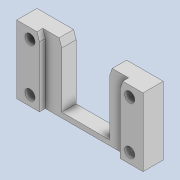
# Autodesk Inventor part: 0008-10-003
Saved by Autodesk Inventor 2020 (Build 240168000, 168)
## iProperties
Created: 2021-02-20
Part Number: 0008-10-003
Material: Generic
Document SubType Name: Modeling
Designer: Iulian Bors
Density: 1 g/cm^3
Appearance: Default
Mass: 4.90136 g
Surface Area: 35.6729 cm^2
Volume: 4.90136 cm^3
Description: Fixare Cap seringa
Author: Iulian Bors
Subject: 003
Autodesk Inventor part; units mm, degrees
ref_plane "YZ Plane" through (0, 0, 0) normal (1, 0, 0) x (0, 1, 0)
ref_plane "XZ Plane" through (0, 0, 0) normal (0, 1, 0) x (-1, 0, 0)
ref_plane "XY Plane" through (0, 0, 0) normal (0, 0, 1) x (1, 0, 0)
sketch "Sketch1" plane through (0, 0, 0) normal (0, 0, 1) x (1, 0, 0)
  line L0 (-25, 13.5) -> (25, 13.5)
  line L1 (25, 13.5) -> (25, -13.5)
  line L2 (25, -13.5) -> (-25, -13.5)
  line L3 (-25, -13.5) -> (-25, 13.5)
  point P0 (0, 0)
  point P1 (0, 13.5)
  point P2 (-25, 0)
  dimension "d0" = 27
  dimension "d1" = 50
  constraints: 8 end point, 2 midpoint, 2 parallel, 1 horizontal, 1 horizontal alignment, 1 perpendicular, 1 vertical alignment
  measures "d0" distance of L2.end L0.start
  measures "d1" distance of L0.start L0.end
extrude "Extrusion1" add sketch "Sketch1" along normal blind 8
sketch "Sketch2" plane through (0, 0, 8) normal (0, 0, 1) x (1, 0, 0)
  arc A0 (-10.3042, 3.1624) -> (-9.6648, 2.3936) centre (-9.9845, 2.778) ccw
  line L0 (-1.0786, 10.8363) -> (-10.3042, 3.1624)
  arc A1 (-0.4391, 10.0675) -> (-1.0786, 10.8363) centre (-0.7589, 10.4519) ccw
  line L1 (-9.6648, 2.3936) -> (-0.4391, 10.0675)
  arc A2 (-9.156, -1.3455) -> (-8.5165, -2.1143) centre (-8.8363, -1.7299) ccw
  line L2 (3.1448, 8.8863) -> (-9.156, -1.3455)
  arc A3 (3.7843, 8.1175) -> (3.1448, 8.8863) centre (3.4646, 8.5019) ccw
  line L3 (-8.5165, -2.1143) -> (3.7843, 8.1175)
  arc A4 (-8.0078, -5.8535) -> (-7.3683, -6.6223) centre (-7.688, -6.2379) ccw
  line L4 (7.3683, 6.9363) -> (-8.0078, -5.8535)
  arc A5 (8.0078, 6.1675) -> (7.3683, 6.9363) centre (7.688, 6.5519) ccw
  line L5 (-7.3683, -6.6223) -> (8.0078, 6.1675)
  arc A6 (-3.7843, -7.8035) -> (-3.1448, -8.5723) centre (-3.4646, -8.1879) ccw
  line L6 (8.5165, 2.4283) -> (-3.7843, -7.8035)
  arc A7 (9.156, 1.6595) -> (8.5165, 2.4283) centre (8.8363, 2.0439) ccw
  line L7 (-3.1448, -8.5723) -> (9.156, 1.6595)
  arc A8 (0.4391, -9.7535) -> (1.0786, -10.5223) centre (0.7589, -10.1379) ccw
  line L8 (9.6648, -2.0796) -> (0.4391, -9.7535)
  arc A9 (10.3042, -2.8484) -> (9.6648, -2.0796) centre (9.9845, -2.464) ccw
  line L9 (1.0786, -10.5223) -> (10.3042, -2.8484)
  line L10 (9.5, 13.5) -> (-9.5, 13.5)
  line L11 (-9.5, 13.5) -> (-9.5, -11.5)
  line L12 (-9.5, -11.5) -> (9.5, -11.5)
  line L13 (9.5, -11.5) -> (9.5, 13.5)
  line L14 (-25, -13.5) -> (25, -13.5) projected
  line L15 (25, 13.5) -> (-25, 13.5) projected
  point P0 (0, 0)
  point P1 (0, -11.5)
  point P2 (0, -13.5)
  dimension "d4" = 19
  dimension "d5" = 2
  constraints: 28 end point, 20 point on circle, 10 centre point, 2 midpoint, 2 parallel, 1 collinear, 1 horizontal, 1 perpendicular, 1 vertical alignment, 50 other
  measures "d4" distance between parallel lines of L11 L13
  measures "d5" distance between parallel lines of L14 L12
extrude "Extrusion2" cut sketch "Sketch2" against normal through all contours L11 L10 L13 L8 A8 L9 L12 L1 A1 L0 | L0 A1 L1 L11 | L13 L9 A8 L8 | L2 A3 L3 A2 | L4 A5 L5 A4 | L6 A7 L7 A6
sketch "Sketch3" plane through (0, 0, 8) normal (0, 0, 1) x (1, 0, 0)
  line L0 (9.5, 13.5) -> (9.5, -11.5) projected
  line L1 (9.5, -11.5) -> (-9.5, -11.5) projected
  line L2 (-9.5, -11.5) -> (-9.5, 13.5) projected
  line L3 (9.5, 13.5) -> (16, 13.5)
  line L4 (25, 13.5) -> (9.5, 13.5) projected
  line L5 (16, 13.5) -> (16, -16.5)
  line L6 (16, -16.5) -> (-16, -16.5)
  line L7 (-16, -16.5) -> (-16, 13.5)
  line L8 (-9.5, 13.5) -> (-25, 13.5) projected
  circle A0 centre (0, 0.157) radius 12.5 projected
  point P0 (0, 0)
  dimension "d8" = 6.5
  dimension "d9" = 6.5
  dimension "d10" = 5
  constraints: 8 end point, 2 perpendicular, 2 point on line, 1 vertical
  measures "d8" distance between parallel lines of L0 L5
  measures "d9" distance between parallel lines of L2 L7
  measures "d10" distance between parallel lines of L1 L6
extrude "Extrusion3" cut sketch "Sketch3" against normal blind 2.3 contours L3 L5 L6 L7 L8 L2 A0 L1 L0 | A0 L0 | L2 A0 | A0 L1
sketch "Sketch4" plane through (0, 0, 0) normal (0, 0, -1) x (-1, 0, 0)
  line L0 (-25, -13.5) -> (-25, 13.5) projected
  line L1 (-25, 13.5) -> (-9.5, 13.5) projected
  line L2 (25, -13.5) -> (-25, -13.5) projected
  point P0 (0, 0)
  point P1 (-19.75, 9.5)
  point P2 (-19.75, -9.5)
  dimension "d13" = 5.25
  dimension "d14" = 4
  dimension "d15" = 4
  constraints: 1 vertical alignment
  measures "d13" distance from line of L0 point (-19.75, 9.5)
  measures "d14" distance from line of point (-19.75, 9.5) L1
  measures "d15" distance from line of L2 point (-19.75, -9.5)
hole "Hole1" at (19.75, 9.5, 0) at (19.75, -9.5, 0) direction (0, 0, 1) diameter 4 depth 8 tip angle 118 counterbore diameter 7 counterbore depth 3
mirror "Mirror1" about plane through (0, 0, 0) normal (1, 0, 0) of "Hole1"
chamfer "Chamfer1" distance 1 distance2 3 1 edges at (9.5, 13.5, 2.85) measured on face at (16.8333, 13.5, 1.9)
chamfer "Chamfer2" distance 1 distance2 3 1 edges at (16, 13.5, 6.85) measured on face at (17.1667, 13.5, 1.9)
chamfer "Chamfer3" distance 1 distance2 3 1 edges at (-9.5, 13.5, 2.85) measured on face at (-16.8333, 13.5, 1.9)
chamfer "Chamfer4" distance 1 distance2 3 1 edges at (-16, 13.5, 6.85) measured on face at (-17.1667, 13.5, 1.9)
equation "\"d9\" = d8"
body "Solid1"
